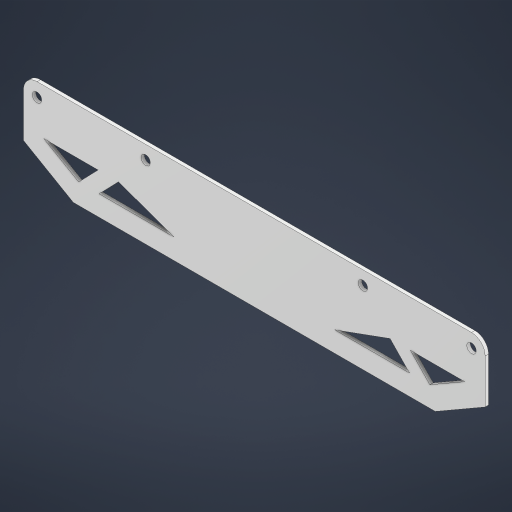
# Autodesk Inventor part: wedge
Saved by Autodesk Inventor 2024 (Build 280153000, 153)
## iProperties
Created: 2023-11-21
Part Number: wedge
Material: Acetal Resin, White
Document SubType Name: Sheet Metal
Designer: avere
Density: 1.425 g/cm^3
Appearance: Smooth - White
Flat Pattern Width: 4.04346 cm
Flat Pattern Length: 21.59 cm
Flat Pattern Area: 87.2982 cm^2
Sheet Metal Rule: Default_mm
Sheet Metal Width: 1.592 in
Sheet Metal Length: 8.500 in
Sheet Metal Area: 13.531 in^2
Author: avere
Autodesk Inventor part; units mm, degrees
ref_plane "YZ Plane" through (0, 0, 0) normal (1, 0, 0) x (0, 1, 0)
ref_plane "XZ Plane" through (0, 0, 0) normal (0, 1, 0) x (-1, 0, 0)
ref_plane "XY Plane" through (0, 0, 0) normal (0, 0, 1) x (1, 0, 0)
sketch "Block1" plane through (0, 0, 0) normal (0, 0, 1) x (1, 0, 0)
  line L0 (-105.9874, 21.1634) -> (-105.9874, 0.5259)
  line L1 (109.9126, 13.2259) -> (-105.9874, 13.2259)
  line L2 (109.9126, 0.5259) -> (109.9126, 21.1634)
  circle A0 centre (-99.6374, 21.1634) radius 2.1844
  arc A1 (-99.6374, 27.5134) -> (-105.9874, 21.1634) centre (-99.6374, 21.1634) ccw
  circle A2 centre (103.5626, 21.1634) radius 2.1844
  arc A3 (109.9126, 21.1634) -> (103.5626, 27.5134) centre (103.5626, 21.1634) ccw
  line L3 (103.5626, 27.5134) -> (-99.6374, 27.5134)
  circle A4 centre (-48.8374, 21.1634) radius 2.1844
  circle A5 centre (52.7626, 21.1634) radius 2.1844
  line L4 (86.6216, -12.9211) -> (-82.6964, -12.9211)
  line L5 (-105.9874, 0.5259) -> (-82.6964, -12.9211)
  line L6 (-105.9874, 0.5259) -> (-79.0933, 0.5259) construction
  line L7 (109.9126, 0.5259) -> (86.6216, -12.9211)
  line L8 (109.9126, 0.5259) -> (136.8067, 0.5259) construction
  line L9 (84.0694, -3.3961) -> (100.3876, 6.0252)
  line L10 (-96.4572, 6.0222) -> (-80.1442, -3.3961)
  line L11 (-80.1442, -3.3961) -> (-71.0624, 6.0222)
  line L12 (-70.6192, -3.3961) -> (-61.5374, 6.0222)
  line L13 (-61.5374, 6.0222) -> (-35.6608, -3.3961)
  line L14 (-71.0624, 6.0222) -> (-96.4572, 6.0222)
  line L15 (74.5444, -3.3961) -> (65.4626, 6.0222)
  line L16 (84.0694, -3.3961) -> (74.9876, 6.0222)
  line L17 (84.0694, -3.3961) -> (99.4401, -3.3961) construction
  line L18 (100.3876, 6.0222) -> (74.9876, 6.0222)
  line L19 (65.4626, 6.0222) -> (39.586, -3.3961)
  line L20 (65.4626, 6.0222) -> (92.9999, 6.0222) construction
  line L21 (-70.6192, -3.3961) -> (-35.6608, -3.3961)
  line L22 (39.586, -3.3961) -> (74.5444, -3.3961)
  point P0 (3.9065, 11.282)
  dimension "d16" = 4.3688
  dimension "d17" = 12.7
  dimension "d18" = 4.3688
  dimension "d19" = 12.7
  dimension "d20" = 4.3688
  dimension "d21" = 4.3688
  dimension "d22" = 30
  dimension "d23" = 150
  dimension "d25" = 9.525
  dimension "d28" = 133.958
  dimension "d29" = 200
  measures "d16" diameter of A0
  measures "d17" diameter of A1
  measures "d18" diameter of A2
  measures "d19" diameter of A3
  measures "d20" diameter of A4
  measures "d21" diameter of A5
  measures "d22" angle of L5 L6
  measures "d23" angle of L7 L8
  measures "d25" distance of L12.start L10.end
  measures "d28" angle of L17 L16
sketch "Sketch1" plane through (0, 0, 0) normal (0, 0, 1) x (1, 0, 0)
  line L0 (-6.35, 1.5875) -> (-6.35, -19.05)
  line L1 (209.55, -6.35) -> (-6.35, -6.35)
  line L2 (209.55, -19.05) -> (209.55, 1.5875)
  circle A0 centre (0, 1.5875) radius 2.1844
  arc A1 (0, 7.9375) -> (-6.35, 1.5875) centre (0, 1.5875) ccw
  circle A2 centre (203.2, 1.5875) radius 2.1844
  arc A3 (209.55, 1.5875) -> (203.2, 7.9375) centre (203.2, 1.5875) ccw
  line L3 (203.2, 7.9375) -> (0, 7.9375)
  circle A4 centre (50.8, 1.5875) radius 2.1844
  circle A5 centre (152.4, 1.5875) radius 2.1844
  line L4 (186.259, -32.4971) -> (16.941, -32.4971)
  line L5 (-6.35, -19.05) -> (16.941, -32.4971)
  line L6 (-6.35, -19.05) -> (20.5441, -19.05) construction
  line L7 (209.55, -19.05) -> (186.259, -32.4971)
  line L8 (209.55, -19.05) -> (236.4441, -19.05) construction
  line L9 (183.7068, -22.9721) -> (200.025, -13.5507)
  line L10 (3.1802, -13.5537) -> (19.4932, -22.9721)
  line L11 (19.4932, -22.9721) -> (28.575, -13.5537)
  line L12 (29.0182, -22.9721) -> (38.1, -13.5537)
  line L13 (38.1, -13.5537) -> (63.9766, -22.9721)
  line L14 (28.575, -13.5537) -> (3.1802, -13.5537)
  line L15 (174.1818, -22.9721) -> (165.1, -13.5537)
  line L16 (183.7068, -22.9721) -> (174.625, -13.5537)
  line L17 (183.7068, -22.9721) -> (199.0775, -22.9721) construction
  line L18 (200.025, -13.5537) -> (174.625, -13.5537)
  line L19 (165.1, -13.5537) -> (139.2234, -22.9721)
  line L20 (165.1, -13.5537) -> (192.6373, -13.5537) construction
  line L21 (29.0182, -22.9721) -> (63.9766, -22.9721)
  line L22 (139.2234, -22.9721) -> (174.1818, -22.9721)
  point P0 (0, 0)
  point P1 (200.0198, -13.5537)
extrude "Extrusion1" add sketch "Sketch1" along normal blind 1.5875
feature "Bend Part1" [suppressed]
equation "\"BendRadius\" = Thickness"
equation "\"BendReliefWidth\" = Thickness"
equation "\"BendReliefDepth\" = 0.5 * Thickness"
equation "\"CornerReliefSize\" = 4 * Thickness"
equation "\"MinimumRemnant\" = 2 * Thickness"
equation "\"TransitionRadius\" = BendRadius"
equation "\"JacobiRadiusSize\" = BendRadius"
equation "\"GapSize\" = Thickness"
equation "\"Thickness\" = 1.5875"
body "Solid1"
